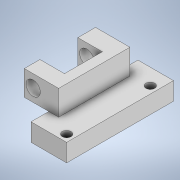
# Autodesk Inventor part: test hålare
Saved by Autodesk Inventor 2022.1 (Build 261234020, 234B)
## iProperties
Created: 2021-11-05
Part Number: test hålare
Material: Generic
Document SubType Name: Modeling
Designer: 46734
Density: 1 g/cm^3
Appearance: Default
Author: 46734
## iProperties of the stored document test hålare_3DPrint.ipt
Created: 2021-11-05
Part Number: test hålare_3DPrint
Material: Generic
Document SubType Name: Modeling
Designer: 46734
Density: 1 g/cm^3
Appearance: Default
Author: 46734
Autodesk Inventor part; units mm, degrees
ref_plane "YZ Plane" through (0, 0, 0) normal (1, 0, 0) x (0, 1, 0)
ref_plane "XZ Plane" through (0, 0, 0) normal (0, 1, 0) x (-1, 0, 0)
ref_plane "XY Plane" through (0, 0, 0) normal (0, 0, 1) x (1, 0, 0)
sketch "Sketch1" plane through (0, 0, 0) normal (0, 1, 0) x (-1, 0, 0)
  line L0 (0, 0) -> (10, 0)
  line L1 (10, 0) -> (10, -30)
  line L2 (10, -30) -> (0, -30)
  line L3 (0, -30) -> (0, 0)
  dimension "d0" = 30
  dimension "d1" = 10
  constraints: 8 end point, 2 parallel, 1 horizontal, 1 perpendicular
  measures "d0" distance of L0.end L1.end
  measures "d1" distance between parallel lines of L1 L3
extrude "Extrusion1" add sketch "Sketch1" along normal blind 5
sketch "Sketch2" plane through (0, 5, 0) normal (0, 1, 0) x (1, 0, 0)
  circle A0 centre (-2, 2) radius 1.25
  circle A1 centre (-2, 25.4965) radius 1.25
  line L0 (0, 0) -> (0, 30) projected
  line L1 (-10, 0) -> (0, 0) projected
  dimension "d4" = 2.5
  dimension "d5" = 2.5
  dimension "d6" = 23.4965
  dimension "d7" = 2
  dimension "d8" = 2
  constraints: 2 centre point, 1 vertical alignment
  measures "d4" diameter of A0
  measures "d5" diameter of A1
  measures "d6" distance of A1.centre A0.centre
  measures "d7" distance from line of A0.centre L0
  measures "d8" distance from line of L1 A0.centre
extrude "Extrusion2" cut sketch "Sketch2" against normal through all
sketch "Sketch3" plane through (0, 5, 0) normal (0, 1, 0) x (1, 0, 0)
  line L0 (-10, 30) -> (-10, 0) projected
  line L1 (-10, 5) -> (-10, 25)
  line L2 (-10, 25) -> (-16.8813, 25)
  line L3 (-16.8813, 25) -> (-16.8813, 5)
  line L4 (-16.8813, 5) -> (-10, 5)
  line L5 (-7.2371, 5) -> (-7.2371, 25)
  line L6 (-7.2371, 25) -> (-10, 25)
  line L7 (-10, 5) -> (-7.2371, 5)
  line L8 (-10, 0) -> (0, 0) projected
  dimension "d11" = 20
  dimension "d22" = 5
  constraints: 14 end point, 5 perpendicular, 4 point on line, 1 parallel
  measures "d11" distance of L1.start L1.end
  measures "d22" distance between parallel lines of L8 L4
extrude "Extrusion3" add sketch "Sketch3" along normal blind 7
sketch "Sketch4" plane through (-10, 5, -25) normal (0, 0, -1) x (-1, 0, 0)
  circle A0 centre (4.3813, 3.5) radius 2
  line L0 (6.8813, 0) -> (6.8813, 7) projected
  point P0 (-10, -5)
  dimension "d14" = 4
  dimension "d15" = 2.5
  constraints: 1 centre point
  measures "d14" diameter of A0
  measures "d15" distance from line of L0 A0.centre
extrude "Extrusion4" cut sketch "Sketch4" against normal through all
sketch "Sketch5" plane through (0, 12, 0) normal (0, 1, 0) x (1, 0, 0)
  line L0 (-16.8813, 25) -> (-16.8813, 5) projected
  line L1 (-10, 30) -> (-10, 0) projected
  line L2 (-16.8813, 10) -> (-10, 10)
  line L3 (-10, 10) -> (-10, 19.25)
  line L4 (-10, 19.25) -> (-16.8813, 19.25)
  line L5 (-16.8813, 19.25) -> (-16.8813, 10)
  line L6 (-16.8813, 5) -> (-7.2371, 5) projected
  point P0 (0, 0)
  point P1 (-16.8813, 19.25)
  point P2 (-10, 10)
  dimension "d18" = 9.25
  dimension "d19" = 5
  constraints: 8 end point, 2 parallel, 2 point on line, 1 horizontal, 1 perpendicular
  measures "d18" distance of L3.end L2.end
  measures "d19" distance between parallel lines of L6 L2
extrude "Extrusion5" cut sketch "Sketch5" against normal through all contours L4 L1 L2 L0
sketch "Sketch6" plane through (0, 12, 0) normal (0, 1, 0) x (1, 0, 0)
  line L0 (-16.8813, 10) -> (-16.8813, 5) projected
  line L1 (-10, 30) -> (-10, 0) projected
  line L2 (-16.8813, 9.3856) -> (-10, 9.3856)
  line L3 (-10, 9.3856) -> (-10, 20.0346)
  line L4 (-10, 20.0346) -> (-16.8813, 20.0346)
  line L5 (-16.8813, 20.0346) -> (-16.8813, 9.3856)
  point P0 (0, 0)
  constraints: 8 end point, 2 parallel, 2 point on line, 1 horizontal, 1 perpendicular
extrude "Extrusion6" cut sketch "Sketch6" against normal through all
body "Solid1"
